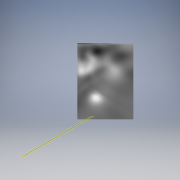
# Autodesk Inventor part: 04_Mirror
Saved by Autodesk Inventor 2016 (Build 200138000, 138)
## iProperties
Created: 2016-11-08
Part Number: 04_Mirror
Material: Generisch
Document SubType Name: Modeling
Designer: Bene
Density: 1 g/cm^3
Appearance: Chrom - poliert
Author: Bene
Autodesk Inventor part; units mm, degrees
ref_plane "YZ Plane" through (0, 0, 0) normal (1, 0, 0) x (0, 1, 0)
ref_plane "XZ Plane" through (0, 0, 0) normal (0, 1, 0) x (-1, 0, 0)
ref_plane "XY Plane" through (0, 0, 0) normal (0, 0, 1) x (1, 0, 0)
ref_plane "Arbeitsebene1" through (0, 141, -63) normal (0, 0, -1) x (-1, 0, 0)
sketch "Skizze1" plane through (0, 141, -63) normal (0, 0, -1) x (-1, 0, 0)
  line L0 (-19.6412, -28.1962) -> (-21.0554, -29.6104)
  line L1 (-21.0554, -29.6104) -> (8.6431, -59.3089)
  line L2 (8.6431, -59.3089) -> (10.0573, -57.8947)
  line L3 (10.0573, -57.8947) -> (-19.6412, -28.1962)
  line L4 (-19.6412, -28.1962) -> (-17.6412, -28.1962) construction
  line L5 (1.1397, -48.9771) -> (46.1397, -48.9771) projected
  line L6 (1.1397, -18.9771) -> (1.1397, -48.9771) projected
  point P0 (0, -141)
  dimension "d0" = 2
  dimension "d1" = 135
  dimension "d2" = 42
  constraints: 10 end point, 2 parallel, 1 equal length, 1 horizontal, 1 perpendicular, 1 point on line
  measures "d0" distance of L0.start L0.end
  measures "d1" angle of L0 L4
  measures "d2" distance of L1.end L0.end
extrude "Extrusion1" add sketch "Skizze1" along normal blind 3 and the other way blind 66
